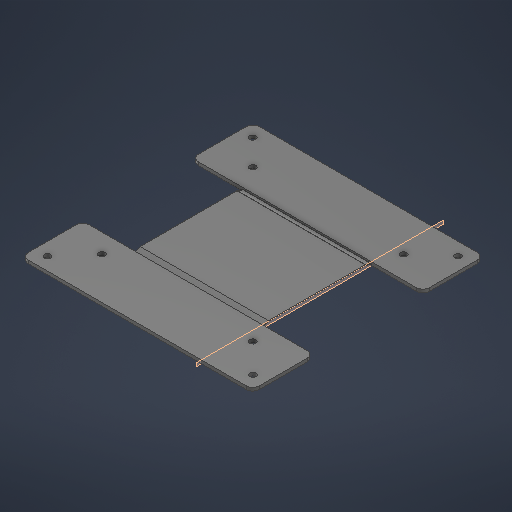
# Autodesk Inventor part: Monitor Base v1.0
Saved by Autodesk Inventor 2027 (Build 310192060, 192F)
## iProperties
Created: 2026-05-19
Part Number: Monitor Base v1.0
Material: Generic
Document SubType Name: Modeling
Designer: cheap
Density: 1 g/cm^3
Appearance: Default
Author: cheap
Autodesk Inventor part; units mm, degrees
ref_plane "XZ Plane" through (0, 0, 0) normal (0, 1, 0) x (-1, 0, 0)
ref_plane "XY Plane" through (0, 0, 0) normal (0, 0, 1) x (1, 0, 0)
sketch "Sketch1" plane through (0, 0, 0) normal (0, 1, 0) x (-1, 0, 0)
  line L0 (3.175, 0) -> (111.125, 0)
  line L1 (114.3, 3.175) -> (114.3, 26.9875)
  line L2 (111.125, 30.1625) -> (92.075, 30.1625)
  line L3 (92.075, 84.1375) -> (111.125, 84.1375)
  line L4 (114.3, 87.3125) -> (114.3, 111.125)
  line L5 (111.125, 114.3) -> (3.175, 114.3)
  line L6 (0, 111.125) -> (0, 87.3125)
  line L7 (3.175, 84.1375) -> (22.225, 84.1375)
  line L8 (22.225, 30.1625) -> (3.175, 30.1625)
  line L9 (0, 3.175) -> (0, 26.9875)
  arc A0 (114.3, 111.125) -> (111.125, 114.3) centre (111.125, 111.125) ccw
  arc A1 (111.125, 84.1375) -> (114.3, 87.3125) centre (111.125, 87.3125) ccw
  arc A2 (114.3, 26.9875) -> (111.125, 30.1625) centre (111.125, 26.9875) ccw
  arc A3 (111.125, 0) -> (114.3, 3.175) centre (111.125, 3.175) ccw
  arc A4 (0, 3.175) -> (3.175, 0) centre (3.175, 3.175) ccw
  arc A5 (3.175, 30.1625) -> (0, 26.9875) centre (3.175, 26.9875) ccw
  arc A6 (0, 87.3125) -> (3.175, 84.1375) centre (3.175, 87.3125) ccw
  arc A7 (3.175, 114.3) -> (0, 111.125) centre (3.175, 111.125) ccw
  line L10 (92.075, 84.1375) -> (22.225, 84.1375)
  line L11 (92.075, 30.1625) -> (22.225, 30.1625)
  point P0 (0, 0)
  point P1 (114.3, 0)
  point P2 (114.3, 30.1625)
  point P3 (88.9, 30.1625)
  point P4 (88.9, 84.1375)
  point P5 (114.3, 84.1375)
  point P6 (114.3, 114.3)
  point P7 (0, 114.3)
  point P8 (0, 84.1375)
  point P9 (25.4, 84.1375)
  point P10 (25.4, 30.1625)
  point P11 (0, 30.1625)
  dimension "d0" = 114.3
  dimension "d1" = 30.1625
  dimension "d2" = 25.4
  dimension "d4" = 30.1625
  dimension "d5" = 114.3
  dimension "d6" = 25.4
  dimension "d9" = 3.175
  dimension "d42" = 114.3
  constraints: 27 point on line, 24 end point, 16 point on circle, 16 tangent, 8 centre point, 4 equal radius, 3 perpendicular, 1 collinear, 1 horizontal, 1 parallel, 1 vertical
  measures "d0" distance of point (0, 0) point (114.3, 0)
  measures "d1" distance of point (114.3, 0) point (114.3, 30.162)
  measures "d2" distance of point (114.3, 30.162) point (88.9, 30.162)
  measures "d4" distance of point (114.3, 84.138) point (114.3, 114.3)
  measures "d5" distance of point (114.3, 114.3) point (0, 114.3)
  measures "d6" distance of point (0, 84.137) point (25.4, 84.137)
  measures "d9" radius of A0
  measures "d42" distance between parallel lines of L5 L0
extrude "Extrusion1" add sketch "Sketch1" along normal blind 1.5875
ref_plane "Work Plane1" through (-25.4, 0, 0) normal (1, 0, 0) x (0, 1, 0)
sketch "Sketch3" plane through (-25.4, 0, 0) normal (1, 0, 0) x (0, 1, 0)
  line L0 (0, 84.1375) -> (1.5875, 84.1375) projected
  line L1 (0.7937, 84.1375) -> (1.8521, 81.1441)
  line L2 (0.7937, 84.1375) -> (3.9688, 84.1375) construction
  line L3 (0, 30.1625) -> (1.5875, 30.1625) construction
  line L4 (7.9375, 57.15) -> (-6.35, 57.15) construction
  line L5 (1.8521, 81.1441) -> (1.8521, 57.15)
  line L6 (0.7938, 30.1625) -> (1.8521, 33.1559)
  line L7 (1.8521, 33.1559) -> (1.8521, 57.15)
  line L8 (0.5015, 30.2658) -> (1.5421, 33.2091)
  line L9 (1.5421, 33.2091) -> (1.5421, 55.5625)
  line L10 (1.5421, 55.5625) -> (1.5421, 81.0909)
  line L11 (1.5421, 81.0909) -> (0.3554, 84.4475)
  line L12 (0.3554, 84.4475) -> (3.9687, 84.4475)
  line L13 (0.5015, 30.2658) -> (0.465, 30.1625)
  line L14 (0.7938, 30.1625) -> (0.465, 30.1625)
  line L15 (0.7937, 84.1375) -> (0.465, 84.1375)
  point P0 (0, 0)
  dimension "d11" = 3.175
  dimension "d12" = 70.529
  constraints: 28 end point, 4 point on line, 2 symmetric about line, 1 collinear, 1 equal length, 1 horizontal, 1 midpoint, 1 perpendicular, 4 other
  measures "d11" distance of L1.start L1.end
  measures "d12" angle of L1 L2
extrude "Extrusion2" add sketch "Sketch3" against normal blind 63.5
sketch "Sketch4" plane through (0, 1.5875, 0) normal (0, 1, 0) x (1, 0, 0)
  circle A0 centre (-107.95, -6.35) radius 1.5875
  line L0 (-111.125, -30.1625) -> (-3.175, -30.1625) projected
  line L1 (-114.3, -3.175) -> (-114.3, -26.9875) projected
  circle A1 centre (-6.35, -6.35) radius 1.5875
  circle A2 centre (-107.95, -107.95) radius 1.5875
  circle A3 centre (-6.35, -107.95) radius 1.5875
  line L2 (-3.175, 0) -> (-111.125, 0) projected
  line L3 (-111.125, -114.3) -> (-3.175, -114.3) projected
  line L4 (-107.95, -6.35) -> (-76.5191, -6.35) construction
  line L5 (-107.95, -6.35) -> (-82.55, -6.35) construction
  circle A4 centre (-95.25, -19.05) radius 1.5875
  circle A5 centre (-20.6375, -19.05) radius 1.5875
  circle A6 centre (-95.25, -93.6625) radius 1.5875
  circle A7 centre (-20.6375, -93.6625) radius 1.5875
  line L6 (0, -26.9875) -> (0, -3.175) projected
  point P0 (0, 0)
  point P1 (-114.3, -15.0812)
  dimension "d15" = 3.175
  dimension "d17" = 6.35
  dimension "d28" = 101.6
  dimension "d31" = 101.6
  dimension "d43" = 107.95
  dimension "d48" = 3.175
  dimension "d51" = 74.6125
  dimension "d54" = 74.6125
  dimension "d57" = 95.25
  dimension "d58" = 95.25
  constraints: 8 centre point, 4 end point, 4 horizontal, 2 vertical, 1 midpoint, 12 other
  measures "d15" diameter of A0
  measures "d17" horizontal distance of point (-114.3, -15.081) L4.start
  measures "d28" distance of L4.start A1.centre
  measures "d31" distance of L4.start A2.centre
  measures "d43" distance from line of L3 L4.start
  measures "d48" diameter of A4
  measures "d51" distance of A4.centre A5.centre
  measures "d54" distance of A4.centre A6.centre
  measures "d57" distance from line of L6 A4.centre
  measures "d58" distance from line of L3 A4.centre
extrude "Extrusion4" cut sketch "Sketch4" against normal blind 63.5
body "Solid1"
